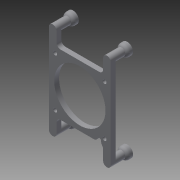
# Autodesk Inventor part: Base
Saved by Autodesk Inventor 2013 (Build 170138000, 138)
## iProperties
Created: 2014-11-16
Part Number: Base
Material: Generic
Document SubType Name: Modeling
Designer: Kyle
Density: 1 g/cm^3
Author: Kyle
Autodesk Inventor part; units mm, degrees
ref_plane "YZ Plane" through (0, 0, 0) normal (1, 0, 0) x (0, 1, 0)
ref_plane "XZ Plane" through (0, 0, 0) normal (0, 1, 0) x (-1, 0, 0)
ref_plane "XY Plane" through (0, 0, 0) normal (0, 0, 1) x (1, 0, 0)
sketch "Sketch1" plane through (0, 0, 0) normal (0, 0, 1) x (1, 0, 0)
  line L0 (0, 0) -> (40.005, 0)
  line L1 (40.005, 0) -> (40.005, -40.005)
  line L2 (40.005, -40.005) -> (0, -40.005)
  line L3 (0, -40.005) -> (0, 0)
  circle A0 centre (3.81, -36.195) radius 1.27
  circle A1 centre (3.81, -3.81) radius 1.27
  circle A2 centre (36.195, -36.195) radius 1.27
  circle A3 centre (36.195, -3.81) radius 1.27
  circle A4 centre (20.0025, -20.0025) radius 16.8275
  point P0 (20.0025, -3.175)
  point P1 (20.0025, -36.83)
  point P2 (36.83, -20.0025)
  point P3 (3.175, -20.0025)
  dimension "d0" = 40.005
  dimension "d1" = 40.005
  dimension "d2" = 3.175
  dimension "d3" = 3.175
  dimension "d4" = 3.175
  dimension "d5" = 3.175
  dimension "d6" = 3.81
  dimension "d7" = 3.81
  dimension "d8" = 3.81
  dimension "d9" = 3.81
  dimension "d10" = 2.54
  dimension "d11" = 2.54
  dimension "d13" = 2.54
  dimension "d14" = 2.54
  constraints: 8 end point, 4 centre point, 4 coincident, 2 parallel, 1 horizontal, 1 horizontal alignment, 1 perpendicular, 2 other
  measures "d0" distance of L0.start L0.end
  measures "d1" distance of L2.end L0.start
  measures "d2" distance from line of L3 point (3.175, -20.002)
  measures "d3" distance from line of L2 point (20.003, -36.83)
  measures "d4" distance from line of L1 point (36.83, -20.002)
  measures "d5" distance from line of L0 point (20.003, -3.175)
  measures "d6" distance from line of L2 point (36.195, -36.195)
  measures "d7" distance from line of point (36.195, -36.195) L1
  measures "d8" distance from line of L0 point (3.81, -3.81)
  measures "d9" distance from line of L3 point (3.81, -3.81)
  measures "d10" diameter of A0
  measures "d11" diameter of A1
  measures "d13" diameter of A2
  measures "d14" diameter of A3
extrude "Extrusion1" add sketch "Sketch1" along normal blind 3.175
sketch "Sketch2" plane through (0, 0, 0) normal (0, 0, -1) x (-1, 0, 0)
  circle A0 centre (-36.195, -3.81) radius 1.27 projected
  circle A1 centre (-36.195, -36.195) radius 1.27 projected
  circle A2 centre (-3.81, -3.81) radius 1.27 projected
  circle A3 centre (-3.81, -36.195) radius 1.27 projected
extrude "Extrusion2" cut sketch "Sketch2" against normal blind 16.51
sketch "Sketch3" plane through (40.005, -40.005, 0) normal (1, 0, 0) x (0, 0, -1)
  line L0 (0, 40.005) -> (0, 0) projected
  line L1 (-3.175, 0) -> (0, 0)
  line L2 (0, 0) -> (0, 5.08)
  line L3 (0, 5.08) -> (-3.175, 5.08)
  line L4 (-3.175, 5.08) -> (-3.175, 0)
  dimension "d22" = 5.08
  constraints: 8 end point, 2 parallel, 1 horizontal, 1 perpendicular, 1 point on line
  measures "d22" distance of L1.end L2.end
extrude "Extrusion3" add sketch "Sketch3" along normal blind 0.3175
sketch "Sketch4" plane through (0, -40.005, 0) normal (-1, 0, 0) x (0, 0, 1)
  line L0 (0, 0) -> (0, 40.005) projected
  line L1 (3.175, 40.005) -> (3.175, 0) projected
  line L2 (0, 0) -> (3.175, 0)
  line L3 (3.175, 0) -> (3.175, 5.08)
  line L4 (0, 5.08) -> (0, 0)
  line L5 (3.175, 40.005) -> (0, 40.005)
  line L6 (0, 40.005) -> (0, 34.925)
  line L7 (3.175, 34.925) -> (3.175, 40.005)
  line L8 (0, 34.925) -> (0, 5.08)
  line L9 (3.175, 5.08) -> (3.175, 34.925)
  dimension "d26" = 5.08
  dimension "d27" = 5.08
  constraints: 16 end point, 2 collinear, 2 horizontal, 2 parallel, 2 perpendicular, 2 point on line
  measures "d26" distance of L4.start L0.start
  measures "d27" distance of L5.end L6.end
extrude "Extrusion4" add sketch "Sketch4" along normal blind 0.3175
sketch "Sketch5" plane through (40.005, 0, 3.175) normal (1, 0, 0) x (0, 0, -1)
  line L0 (0, -34.925) -> (0, 0) projected
  line L1 (3.175, 0) -> (0, 0)
  line L2 (0, 0) -> (0, -5.08)
  line L3 (3.175, -5.08) -> (3.175, 0)
  line L4 (3.175, 0) -> (3.175, -34.925) projected
  line L5 (0, -5.08) -> (0, -34.925)
  line L6 (0, -34.925) -> (3.175, -34.925)
  line L7 (3.175, -34.925) -> (3.175, -5.08)
  dimension "d30" = 5.08
  constraints: 12 end point, 2 collinear, 2 perpendicular, 1 horizontal, 1 parallel, 1 point on line
  measures "d30" distance of L3.start L1.start
extrude "Extrusion5" add sketch "Sketch5" along normal blind 0.3175
sketch "Sketch6" plane through (40.3225, -40.005, 0) normal (0, -1, 0) x (1, 0, 0)
  line L0 (0, 0) -> (-40.64, 0) projected
  line L1 (0, 3.175) -> (-5.08, 3.175)
  line L2 (-5.08, 3.175) -> (-5.08, 0)
  line L3 (-5.08, 0) -> (0, 0)
  line L4 (0, 0) -> (0, 3.175)
  line L5 (-40.64, 3.175) -> (-35.56, 3.175)
  line L6 (-35.56, 3.175) -> (-35.56, 0)
  line L7 (-35.56, 0) -> (-40.64, 0)
  line L8 (-40.64, 0) -> (-40.64, 3.175)
  point P0 (-40.3225, 0)
  dimension "d33" = 5.08
  dimension "d35" = 5.08
  constraints: 16 end point, 4 parallel, 2 horizontal, 2 perpendicular, 2 point on line
  measures "d33" distance of L2.end L3.end
  measures "d35" distance of L0.end L6.end
extrude "Extrusion6" add sketch "Sketch6" along normal blind 11.7475
sketch "Sketch7" plane through (-0.3175, 0, 3.175) normal (0, 1, 0) x (1, 0, 0)
  line L0 (0, 3.175) -> (40.64, 3.175) projected
  line L1 (0, 0) -> (5.08, 0)
  line L2 (5.08, 0) -> (5.08, 3.175)
  line L3 (5.08, 3.175) -> (0, 3.175)
  line L4 (0, 3.175) -> (0, 0)
  line L5 (40.64, 0) -> (35.56, 0)
  line L6 (35.56, 0) -> (35.56, 3.175)
  line L7 (35.56, 3.175) -> (40.64, 3.175)
  line L8 (40.64, 3.175) -> (40.64, 0)
  point P0 (0.3175, 3.175)
  dimension "d38" = 5.08
  dimension "d40" = 5.08
  constraints: 16 end point, 4 parallel, 2 horizontal, 2 perpendicular, 2 point on line
  measures "d38" distance of L6.end L7.end
  measures "d40" distance of L2.end L0.start
extrude "Extrusion7" add sketch "Sketch7" along normal blind 11.7475
fillet "Fillet1" radius 2.54 4 edges at (40.3225, 11.7475, 1.5875) (35.2425, 11.7475, 1.5875) (4.7625, 11.7475, 1.5875) (-0.3175, 11.7475, 1.5875)
fillet "Fillet2" radius 2.54 4 edges at (4.7625, -51.7525, 1.5875) (40.3225, -51.7525, 1.5875) (35.2425, -51.7525, 1.5875) (-0.3175, -51.7525, 1.5875)
fillet "Fillet4" radius 2.54 4 edges at (35.2425, -40.005, 1.5875) (4.7625, -40.005, 1.5875) (4.7625, 0, 1.5875) (35.2425, 0, 1.5875)
sketch "Sketch9" plane through (0, 0, 0) normal (0, 0, -1) x (-1, 0, 0)
  arc A0 (-40.3225, -49.2125) -> (-35.2425, -49.2125) centre (-37.7825, -49.2125) ccw projected
  arc A1 (-4.7625, -49.2125) -> (0.3175, -49.2125) centre (-2.2225, -49.2125) ccw projected
  arc A2 (0.3175, 9.2075) -> (-4.7625, 9.2075) centre (-2.2225, 9.2075) ccw projected
  arc A3 (-35.2425, 9.2075) -> (-40.3225, 9.2075) centre (-37.7825, 9.2075) ccw projected
  circle A4 centre (-37.7825, 9.2075) radius 2.54
  circle A5 centre (-2.2225, 9.2075) radius 2.54
  circle A6 centre (-2.2225, -49.2125) radius 2.54
  circle A7 centre (-37.7825, -49.2125) radius 2.54
  point P0 (0, 0)
  constraints: 4 coincident, 4 horizontal alignment, 8 other
extrude "Extrusion9" add sketch "Sketch9" along normal blind 6.35
sketch "Sketch10" plane through (37.7825, 9.2075, -6.35) normal (0, 0, -1) x (-1, 0, 0)
  circle A0 centre (0, 0) radius 2.54 projected
  circle A1 centre (0, 0) radius 3.81
  point P0 (37.7825, -9.2075)
  dimension "d60" = 7.62
  constraints: 1 centre point, 1 coincident
  measures "d60" diameter of A1
extrude "Extrusion10" add sketch "Sketch10" along normal blind 3.81 contours A0 | A1
sketch "Sketch11" plane through (2.2225, 9.2075, -6.35) normal (0, 0, -1) x (-1, 0, 0)
  circle A0 centre (0, 0) radius 2.54 projected
  circle A1 centre (0, 0) radius 3.81
  point P0 (2.2225, -9.2075)
  dimension "d65" = 7.62
  constraints: 1 centre point, 1 coincident
  measures "d65" diameter of A1
extrude "Extrusion11" add sketch "Sketch11" along normal blind 3.81 contours A0 | A1
sketch "Sketch12" plane through (37.7825, -49.2125, -6.35) normal (0, 0, -1) x (-1, 0, 0)
  circle A0 centre (0, 0) radius 2.54 projected
  circle A1 centre (0, 0) radius 3.81
  point P0 (37.7825, 49.2125)
  dimension "d69" = 7.62
  constraints: 1 centre point, 1 coincident
  measures "d69" diameter of A1
extrude "Extrusion12" add sketch "Sketch12" along normal blind 3.81 contours A0 | A1
sketch "Sketch13" plane through (2.2225, -49.2125, -6.35) normal (0, 0, -1) x (-1, 0, 0)
  circle A0 centre (0, 0) radius 2.54 projected
  circle A1 centre (0, 0) radius 3.81
  point P0 (2.2225, 49.2125)
  dimension "d73" = 7.62
  constraints: 1 centre point, 1 coincident
  measures "d73" diameter of A1
extrude "Extrusion13" add sketch "Sketch13" along normal blind 3.81 contours A0 | A1
fillet "Fillet5" radius 2.54 1 edges at (41.5925, -49.2125, -6.35)
fillet "Fillet6" radius 2.54 3 edges at (6.0325, -49.2125, -6.35) (6.0325, 9.2075, -6.35) (41.5925, 9.2075, -6.35)
sketch "Sketch18" plane through (0, 0, 0) normal (0, 0, -1) x (-1, 0, 0)
  line L0 (-32.7025, -40.005) -> (-7.3025, -40.005) projected
  line L1 (-40.3225, 9.2075) -> (-40.3225, -49.2125) projected
  arc A0 (-32.7025, -40.005) -> (-35.2425, -42.545) centre (-32.7025, -42.545) ccw projected
  arc A1 (-31.4325, -38.735) -> (-33.9725, -38.735) centre (-32.7025, -38.735) ccw
  line L2 (-31.4325, -40.005) -> (-31.4325, -38.735)
  line L3 (-33.9725, -38.735) -> (-33.9725, -40.3453)
  point P0 (0, 0)
  dimension "d101" = 1.27
  dimension "d102" = 7.62
  constraints: 4 end point, 4 point on circle, 2 tangent, 1 centre point, 1 coincident, 1 parallel, 1 point on line
  measures "d101" distance from line of point (-32.702, -38.735) L0
  measures "d102" distance from line of point (-32.702, -38.735) L1
extrude "Extrusion18" cut sketch "Sketch18" against normal blind 12.7
fillet "Fillet8" radius 2.54 1 edges at (33.9725, -40.3453, 1.5875)
fillet "Fillet9" radius 2.54 1 edges at (31.4325, -40.005, 1.5875)
sketch "Sketch19" plane through (37.7825, 9.2075, -10.16) normal (0, 0, -1) x (-1, 0, 0)
  circle A0 centre (0, 0) radius 3.81 projected
  circle A1 centre (0, 0) radius 1.27
  circle A2 centre (35.56, 0) radius 1.27
  circle A3 centre (35.56, -58.42) radius 1.27
  circle A4 centre (0, -58.42) radius 1.27
  point P0 (37.7825, -9.2075)
  dimension "d105" = 2.54
  dimension "d107" = 35.56
  dimension "d108" = 58.42
  constraints: 4 centre point, 4 coincident
  measures "d105" diameter of A1
  measures "d107" distance of point (35.56, 0) A0.centre
  measures "d108" vertical distance of point (35.56, -58.42) A0.centre
extrude "Extrusion19" cut sketch "Sketch19" against normal blind 7.62 contours A1 | A2 | A3 | A4
body "Solid1"
